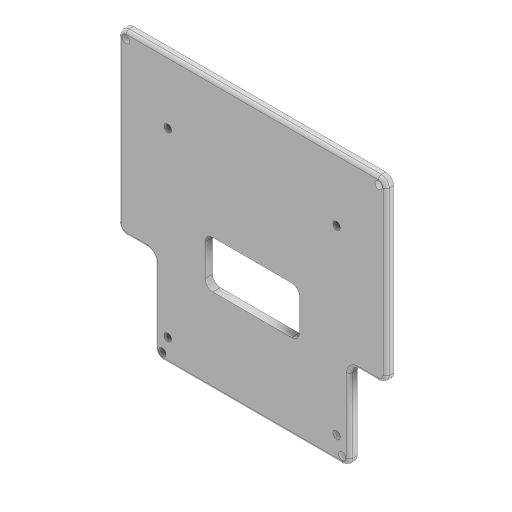
# Autodesk Inventor part: bit bot lid 1
Saved by Autodesk Inventor 2024 (Build 280153000, 153)
## iProperties
Created: 2024-01-27
Part Number: bit bot lid 1
Material: Generic
Document SubType Name: Modeling
Designer: chris
Density: 1 g/cm^3
Appearance: Default
Author: chris
Autodesk Inventor part; units mm, degrees
ref_plane "YZ Plane" through (0, 0, 0) normal (1, 0, 0) x (0, 1, 0)
ref_plane "XZ Plane" through (0, 0, 0) normal (0, 1, 0) x (-1, 0, 0)
ref_plane "XY Plane" through (0, 0, 0) normal (0, 0, 1) x (1, 0, 0)
sketch "Sketch1" plane through (0, 0, 0) normal (0, 0, 1) x (1, 0, 0)
  arc A0 (-50.8, 107.95) -> (-53.975, 104.775) centre (-50.8, 104.775) ccw
  line L0 (-53.975, 104.775) -> (-53.975, 39.4462)
  arc A1 (-53.975, 39.4462) -> (-50.8, 36.2712) centre (-50.8, 39.4462) ccw
  line L1 (-50.8, 36.2712) -> (-42.4561, 36.2712)
  arc A2 (-39.2811, 33.0962) -> (-42.4561, 36.2712) centre (-42.4561, 33.0962) ccw
  line L2 (-39.2811, 33.0962) -> (-39.2811, 3.175)
  arc A3 (-39.2811, 3.175) -> (-36.1061, 0) centre (-36.1061, 3.175) ccw
  line L3 (-36.1061, 0) -> (36.1061, 0)
  arc A4 (36.1061, 0) -> (39.2811, 3.175) centre (36.1061, 3.175) ccw
  line L4 (39.2811, 3.175) -> (39.2811, 33.0962)
  arc A5 (42.4561, 36.2712) -> (39.2811, 33.0962) centre (42.4561, 33.0962) ccw
  line L5 (42.4561, 36.2712) -> (50.8, 36.2712)
  arc A6 (50.8, 36.2712) -> (53.975, 39.4462) centre (50.8, 39.4462) ccw
  line L6 (53.975, 39.4462) -> (53.975, 104.775)
  arc A7 (53.975, 104.775) -> (50.8, 107.95) centre (50.8, 104.775) ccw
  line L7 (50.8, 107.95) -> (-50.8, 107.95)
  arc A8 (39.4081, 39.3192) -> (36.2331, 36.1442) centre (39.4081, 36.1442) ccw
  line L8 (36.2331, 36.1442) -> (36.2331, 9.271)
  arc A9 (33.0581, 6.096) -> (36.2331, 9.271) centre (33.0581, 9.271) ccw
  line L9 (33.0581, 6.096) -> (-33.0581, 6.096)
  arc A10 (-36.2331, 9.271) -> (-33.0581, 6.096) centre (-33.0581, 9.271) ccw
  line L10 (-36.2331, 9.271) -> (-36.2331, 36.1442)
  arc A11 (-36.2331, 36.1442) -> (-39.4081, 39.3192) centre (-39.4081, 36.1442) ccw
  line L11 (-39.4081, 39.3192) -> (-47.752, 39.3192)
  arc A12 (-50.927, 42.4942) -> (-47.752, 39.3192) centre (-47.752, 42.4942) ccw
  line L12 (-50.927, 42.4942) -> (-50.927, 98.679)
  arc A13 (-47.752, 101.854) -> (-50.927, 98.679) centre (-47.752, 98.679) ccw
  line L13 (-47.752, 101.854) -> (47.752, 101.854)
  arc A14 (50.927, 98.679) -> (47.752, 101.854) centre (47.752, 98.679) ccw
  line L14 (50.927, 98.679) -> (50.927, 42.4942)
  arc A15 (47.752, 39.3192) -> (50.927, 42.4942) centre (47.752, 42.4942) ccw
  line L15 (47.752, 39.3192) -> (39.4081, 39.3192)
  circle A16 centre (-50.927, 104.902) radius 1.5
  circle A17 centre (36.2331, 3.048) radius 1.5
  circle A18 centre (-36.2331, 3.048) radius 1.5
  circle A19 centre (50.927, 104.902) radius 1.5
  line L16 (0, 0) -> (0, -19.0308)
  constraints: 34 end point, 32 point on circle, 20 centre point, 1 vertical
extrude "Extrusion1" add sketch "Sketch1" along normal blind 3 contours L7 A7 L6 A6 L5 A5 L4 A4 L3 A3 L2 A2 L1 A1 L0 A0 | A8 L8 A9 L9 A10 L10 A11 L11 A12 L12 A13 L13 A14 L14 A15 L15
fillet "Fillet1" radius 1.25 16 edges at (53.0451, 107.0201, 3) (0, 107.95, 3) (-53.0451, 107.0201, 3) (-53.975, 72.1106, 3) (-53.0451, 37.2011, 3) (-46.6281, 36.2712, 3) (-40.211, 35.3413, 3) (-39.2811, 18.1356, 3) (-38.3512, 0.9299, 3) (0, 0, 3) (38.3512, 0.9299, 3) (39.2811, 18.1356, 3) (40.211, 35.3413, 3) (46.6281, 36.2712, 3) (53.0451, 37.2011, 3) (53.975, 72.1106, 3)
sketch "Sketch2" plane through (0, 0, 3) normal (0, 0, 1) x (1, 0, 0)
  arc A0 (-30.9142, 9.83) -> (-32.3284, 10.83) centre (-32.3284, 9.33) ccw
  line L0 (-32.5, 10.83) -> (-32.3284, 10.83)
  line L1 (-32.5, 80.83) -> (-32.5, 10.83)
  line L2 (32.5, 80.83) -> (-32.5, 80.83)
  line L3 (32.5, 10.83) -> (32.5, 80.83)
  line L4 (32.3284, 10.83) -> (32.5, 10.83)
  arc A1 (32.3284, 10.83) -> (30.9142, 9.83) centre (32.3284, 9.33) ccw
  arc A2 (29.5, 8.83) -> (30.9142, 9.83) centre (29.5, 10.33) ccw
  line L5 (29.5, 8.83) -> (-29.5, 8.83)
  arc A3 (-30.9142, 9.83) -> (-29.5, 8.83) centre (-29.5, 10.33) ccw
  arc A4 (-35, 85.33) -> (-37, 83.33) centre (-35, 83.33) ccw
  line L6 (-37, 8.33) -> (-37, 83.33)
  arc A5 (-37, 8.33) -> (-35, 6.33) centre (-35, 8.33) ccw
  line L7 (35, 6.33) -> (-35, 6.33)
  arc A6 (35, 6.33) -> (37, 8.33) centre (35, 8.33) ccw
  line L8 (37, 83.33) -> (37, 8.33)
  arc A7 (37, 83.33) -> (35, 85.33) centre (35, 83.33) ccw
  line L9 (-35, 85.33) -> (35, 85.33)
  circle A8 centre (34, 82.33) radius 1.5
  circle A9 centre (-34, 82.33) radius 1.5
  circle A10 centre (-34, 9.33) radius 1.5
  circle A11 centre (34, 9.33) radius 1.5
  line L10 (36.1061, 1.25) -> (-36.1061, 1.25) projected
  line L11 (0, 6.33) -> (0, -2.8147)
  line L12 (0, 1.25) -> (0, 6.33)
  line L13 (0, 8.83) -> (0, 34.23)
  line L14 (0, 34.23) -> (-19.05, 34.23)
  line L15 (-19.05, 34.23) -> (-19.05, 53.28)
  line L16 (-19.05, 53.28) -> (19.05, 53.28)
  line L17 (19.05, 53.28) -> (19.05, 34.23)
  line L18 (19.05, 34.23) -> (0, 34.23)
  point P0 (0, 0)
  point P1 (0, 67.33)
  dimension "d4" = 5.08
  dimension "d5" = 25.4
  dimension "d6" = 19.05
  dimension "d7" = 19.05
  dimension "d8" = 38.1
  dimension "d9" = 19.05
  constraints: 36 end point, 16 point on circle, 12 centre point, 3 midpoint, 3 perpendicular, 2 vertical, 1 point on line
  measures "d4" distance of L12.start L12.end
  measures "d5" distance of L13.start L13.end
  measures "d6" distance of L13.end L14.end
  measures "d7" distance of L14.end L15.end
  measures "d8" distance of L15.end L16.end
  measures "d9" distance of L16.end L17.end
extrude "Extrusion2" cut sketch "Sketch2" against normal through all contours L14 L15 L16 L17 L18 | A8 | A9 | A10 | A11
fillet "Fillet2" radius 3.175 4 edges at (-19.05, 53.28, 1.5) (-19.05, 34.23, 1.5) (19.05, 34.23, 1.5) (19.05, 53.28, 1.5)
body "Solid1"
